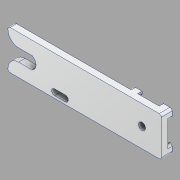
# Autodesk Inventor part: wheel_mount._brake_01ipt
Saved by Autodesk Inventor 2021.3 (Build 253353000, 353)
## iProperties
Created: 2021-07-08
Part Number: wheel_mount._brake_01ipt
Material: アルミニウム 6061
Document SubType Name: Modeling
Designer: gisen
Density: 2.7 g/cm^3
Appearance: アルミニウム - フラット
Author: gisen
Autodesk Inventor part; units mm, degrees
ref_plane "YZ Plane" through (0, 0, 0) normal (1, 0, 0) x (0, 1, 0)
ref_plane "XZ Plane" through (0, 0, 0) normal (0, 1, 0) x (-1, 0, 0)
ref_plane "作業平面1" through (0, 0, 0) normal (0, 0, 1) x (1, 0, 0)
sketch "スケッチ2" plane through (0, 0, 0) normal (0, 0, 1) x (1, 0, 0)
  line L0 (120, -56.75) -> (-20, -56.75)
  line L1 (-20, -56.75) -> (-20, -93.25)
  line L2 (-20, -93.25) -> (120, -93.25)
  line L3 (120, -93.25) -> (120, -56.75)
  circle A0 centre (0, -75) radius 6 construction
  circle A1 centre (0, -75) radius 75 construction
  point P0 (0, 0)
  dimension "d1" = 150
  dimension "d2" = 18.25
  dimension "d3" = 18.25
  dimension "d4" = 20
  dimension "d29" = 120
  constraints: 8 end point, 2 parallel, 1 horizontal, 1 perpendicular, 1 vertical alignment
  measures "d2" distance from line of L0 A0.centre
  measures "d3" distance from line of L2 A0.centre
  measures "d4" distance from line of L1 A0.centre
  measures "d29" distance from line of A0.centre L3
extrude "押し出し1" add sketch "スケッチ2" along normal blind 6
sketch "スケッチ3" plane through (0, 0, 6) normal (0, 0, 1) x (1, 0, 0)
  circle A0 centre (0, -75) radius 6 construction
  circle A1 centre (0, -75) radius 6.25
  line L0 (0, -68.75) -> (-38.1, -68.75) construction
  line L1 (-38.1, -68.75) -> (-38.1, -81.25) construction
  line L2 (-38.1, -81.25) -> (0, -81.25) construction
  line L3 (0, -81.25) -> (0, -68.75) construction
  line L4 (-20, -68) -> (-20, -81.25)
  line L5 (0, -82) -> (0, -68.75)
  line L6 (-20, -56.75) -> (-20, -93.25) projected
  line L7 (-20, -69.25) -> (2.4495, -69.25)
  line L8 (2.4495, -69.25) -> (2.4495, -80.75)
  line L9 (2.4495, -80.75) -> (-20, -80.75)
  line L10 (-20, -80.75) -> (-20, -69.25)
  point P0 (0, 0)
  point P1 (-2.4495, -80.75)
  point P2 (-2.4495, -69.25)
  point P3 (0, -80.75)
  point P4 (0, -69.25)
  point P5 (0, -81.25)
  dimension "d8" = 12.5
  dimension "d30" = 11.5
  constraints: 20 end point, 5 parallel, 3 point on circle, 2 horizontal, 2 perpendicular, 2 point on line, 2 tangent, 1 centre point, 1 coincident, 1 collinear
  measures "d8" diameter of A1
  measures "d30" distance between parallel lines of L7 L9
extrude "押し出し2" cut sketch "スケッチ3" against normal blind 12.5 contours A1 L8 | L8 L9 L5 L7 | L5 L9 A1 L7 | A1 L9 L4 L7
fillet "フィレット1" radius 10 2 edges at (-20, -80.75, 3) (-20, -69.25, 3)
ref_plane "作業平面2" through (-20, -75, 0) normal (0, -1, 0) x (1, 0, 0)
sketch "スケッチ4" plane through (0, 0, 6) normal (0, 0, 1) x (1, 0, 0)
  line L0 (-20, -93.25) -> (120, -93.25) projected
  line L1 (120, -56.75) -> (-20, -56.75) projected
  line L2 (120, -93.25) -> (120, -56.75) projected
  point P0 (0, 0)
  point P1 (105, -75)
  dimension "d25" = 15
  dimension "d26" = 36.5
  dimension "d27" = 18.25
  measures "d25" distance from line of L2 point (105, -75)
  measures "d26" distance between parallel lines of L0 L1
  measures "d27" distance from line of L1 point (105, -75)
hole "穴1" at (105, -75, 6) direction (0, 0, -1) diameter 6.6 end through all
ref_plane "作業平面3" through (0, -75, 0) normal (0, 0.7071, 0.7071) x (-1, 0, 0)
sketch "スケッチ5" plane through (0, 0, 0) normal (0, 0, 1) x (1, 0, 0)
  circle A0 centre (105, -75) radius 3.3 construction
  arc A1 (-20, -59.25) -> (-10, -69.25) centre (-10, -59.25) ccw construction
  line L0 (-10, -69.25) -> (2.4495, -69.25) construction
  arc A2 (2.4495, -80.75) -> (2.4495, -69.25) centre (0, -75) ccw construction
  line L1 (2.4495, -80.75) -> (-10, -80.75) construction
  arc A3 (-10, -80.75) -> (-20, -90.75) centre (-10, -90.75) ccw construction
  line L2 (-20, -90.75) -> (-20, -93.25) construction
  line L3 (-20, -93.25) -> (120, -93.25) construction
  line L4 (120, -93.25) -> (120, -56.75) construction
  line L5 (120, -56.75) -> (-20, -56.75) construction
  line L6 (-20, -56.75) -> (-20, -59.25) construction
  line L7 (123, -56.75) -> (87, -56.75)
  line L8 (87, -56.75) -> (87, -93.25)
  line L9 (87, -93.25) -> (123, -93.25)
  line L10 (123, -93.25) -> (123, -56.75)
  line L11 (120, -93.25) -> (120, -56.75) projected
  line L12 (90, -90.25) -> (120, -90.25)
  line L13 (120, -90.25) -> (120, -59.75)
  line L14 (120, -59.75) -> (90, -59.75)
  line L15 (90, -59.75) -> (90, -90.25)
  line L16 (90, -90.25) -> (120, -59.75) construction
  line L17 (120, -90.25) -> (90, -59.75) construction
  line L18 (87, -85.25) -> (123, -85.25)
  line L19 (123, -85.25) -> (123, -64.75)
  line L20 (123, -64.75) -> (87, -64.75)
  line L21 (87, -64.75) -> (87, -85.25)
  circle A4 centre (105, -75) radius 3.3 projected
  line L22 (87, -85.25) -> (123, -64.75) construction
  line L23 (123, -85.25) -> (87, -64.75) construction
  line L24 (95, -93.25) -> (115, -93.25)
  line L25 (115, -93.25) -> (115, -56.75)
  line L26 (115, -56.75) -> (95, -56.75)
  line L27 (95, -56.75) -> (95, -93.25)
  line L28 (95, -93.25) -> (115, -56.75) construction
  line L29 (115, -93.25) -> (95, -56.75) construction
  point P0 (0, 0)
  point P1 (95, -93.25)
  point P2 (95, -90.25)
  point P3 (90, -85.25)
  point P4 (95, -59.75)
  point P5 (90, -64.75)
  point P6 (120, -85.25)
  point P7 (115, -90.25)
  point P8 (115, -93.25)
  point P9 (115, -59.75)
  point P10 (120, -64.75)
  dimension "d31" = 3
  dimension "d34" = 30.5
  dimension "d35" = 3
  dimension "d36" = 3
  dimension "d37" = 3
  dimension "d38" = 8
  dimension "d39" = 8
  constraints: 44 end point, 8 parallel, 6 midpoint, 4 horizontal, 4 perpendicular, 3 point on line
  measures "d31" distance between parallel lines of L10 L4
  measures "d34" distance of L13.end L12.end
  measures "d35" distance between parallel lines of L9 L12
  measures "d36" distance between parallel lines of L14 L7
  measures "d37" distance between parallel lines of L15 L8
  measures "d38" distance between parallel lines of L7 L20
  measures "d39" distance between parallel lines of L10 L25
extrude "押し出し3" add sketch "スケッチ5" against normal blind 4 contours L10 L20 L11 L7 | L11 L14 L25 L7 | L10 L9 L11 L18 | L27 L14 L15 L20 L8 L7 | L9 L25 L12 L11 | L18 L15 L12 L27 L9 L8
sketch "スケッチ6" plane through (120, -93.25, 0) normal (1, 0, 0) x (0, 0, -1)
  line L0 (0, 8) -> (0, 28.5) projected
  line L1 (0, 36.5) -> (-6, 36.5) projected
  line L2 (-6, 0) -> (-6, 36.5) projected
  line L3 (0, 0) -> (-6, 0) projected
  line L4 (0, 0) -> (0, 3) projected
  line L5 (0, 3) -> (0, 8) projected
  line L6 (0, 28.5) -> (0, 33.5) projected
  line L7 (0, 33.5) -> (0, 36.5) projected
  point P0 (0, 93.25)
extrude "押し出し4" add sketch "スケッチ6" along normal up to surface (3 mm away)
fillet "フィレット2" radius 2 8 edges at (-20, -56.75, 3) (-20, -93.25, 3) (87, -56.75, -2) (87, -93.25, -2) (87, -64.75, -2) (87, -85.25, -2) (123, -64.75, -2) (123, -85.25, -2)
fillet "フィレット2" radius 0.5 16 edges at (115, -59.75, -2) (120, -64.75, -2) (120, -85.25, -2) (115, -90.25, -2) (95, -59.75, -2) (90, -64.75, -2) (90, -62.25, -4) (92.5, -59.75, -4) (117.5, -59.75, -4) (120, -62.25, -4) (120, -87.75, -4) (117.5, -90.25, -4) (95, -90.25, -2) (90, -85.25, -2) (90, -87.75, -4) (92.5, -90.25, -4)
sketch "スケッチ7" plane through (20.6125, 13, 6) normal (0, 0, 1) x (1, 0, 0)
  arc A0 (3.9922, -80.75) -> (-0.2106, -72.4528) centre (-20.6125, -88) ccw
  circle A1 centre (-20.6125, -88) radius 31.5 construction
  circle A2 centre (7.9653, -101.25) radius 2.75 construction
  line L0 (-18, -106.25) -> (105, -106.25) construction
  arc A3 (-18.163, -93.75) -> (-18.163, -82.25) centre (-20.6125, -88) ccw projected
  line L1 (-38.6125, -106.25) -> (100.3875, -106.25) projected
  point P0 (0, 0)
  dimension "d48" = 63
  dimension "d46" = 5.5
  dimension "d47" = 5
  constraints: 3 coincident, 2 centre point, 2 end point, 2 point on circle, 1 collinear, 3 other
  measures "d46" diameter of A2
  measures "d47" distance from line of L0 A2.centre
hole "穴2" at (28.5777, -88.25, 6) direction (0, 0, -1) diameter 5.5 end through all
sketch "スケッチ8" plane through (0, 0, 6) normal (0, 0, 1) x (1, 0, 0)
  circle A0 centre (28.5777, -88.25) radius 2.75 construction
  arc A1 (121, -93.25) -> (123, -91.25) centre (121, -91.25) ccw construction
  line L0 (123, -91.25) -> (123, -58.75) construction
  arc A2 (123, -58.75) -> (121, -56.75) centre (121, -58.75) ccw construction
  line L1 (-18, -56.75) -> (121, -56.75) construction
  arc A3 (-18, -56.75) -> (-20, -58.75) centre (-18, -58.75) ccw construction
  line L2 (-20, -58.75) -> (-20, -59.25) construction
  arc A4 (-20, -59.25) -> (-10, -69.25) centre (-10, -59.25) ccw construction
  line L3 (-10, -69.25) -> (2.4495, -69.25) construction
  arc A5 (2.4495, -80.75) -> (2.4495, -69.25) centre (0, -75) ccw construction
  line L4 (2.4495, -80.75) -> (-10, -80.75) construction
  arc A6 (-10, -80.75) -> (-20, -90.75) centre (-10, -90.75) ccw construction
  line L5 (-20, -90.75) -> (-20, -91.25) construction
  arc A7 (-20, -91.25) -> (-18, -93.25) centre (-18, -91.25) ccw construction
  line L6 (-18, -93.25) -> (121, -93.25) construction
  circle A8 centre (105, -75) radius 3.3 construction
  line L7 (23.5777, -91) -> (33.5777, -91)
  line L8 (33.5777, -91) -> (33.5777, -85.5) construction
  line L9 (33.5777, -85.5) -> (23.5777, -85.5)
  line L10 (23.5777, -85.5) -> (23.5777, -91) construction
  circle A9 centre (28.5777, -88.25) radius 2.75 projected
  line L11 (23.5777, -91) -> (33.5777, -85.5) construction
  line L12 (33.5777, -91) -> (23.5777, -85.5) construction
  arc A10 (33.5777, -91) -> (33.5777, -85.5) centre (33.5777, -88.25) ccw
  arc A11 (23.5777, -85.5) -> (23.5777, -91) centre (23.5777, -88.25) ccw
  point P0 (0, 0)
  dimension "d55" = 10
  constraints: 12 end point, 4 midpoint, 4 point on circle, 2 centre point, 2 parallel, 1 horizontal, 1 perpendicular, 1 tangent
  measures "d55" distance of L9.end L8.end
extrude "押し出し5" cut sketch "スケッチ8" against normal through all
equation "\"d3\" = d2"
equation "\"d9\" = d8"
equation "\"d27\" = 0.5 * d26"
equation "\"d35\" = d31"
equation "\"d36\" = d31"
equation "\"d37\" = d31"
equation "\"d39\" = d38"
